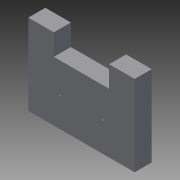
# Autodesk Inventor part: PCB_kon_drzak
Saved by Autodesk Inventor 2015 (Build 190159000, 159)
## iProperties
Created: 2015-12-17
Part Number: PCB_kon_drzak
Material: Generic
Document SubType Name: Modeling
Designer: Turboslimak
Density: 1 g/cm^3
Appearance: Default
Author: Turboslimak
Autodesk Inventor part; units mm, degrees
ref_plane "YZ Plane" through (0, 0, 0) normal (1, 0, 0) x (0, 1, 0)
ref_plane "XZ Plane" through (0, 0, 0) normal (0, 1, 0) x (-1, 0, 0)
ref_plane "XY Plane" through (0, 0, 0) normal (0, 0, 1) x (1, 0, 0)
sketch "Sketch1" plane through (0, 0, 0) normal (0, 1, 0) x (-1, 0, 0)
  line L0 (6.25, 4.75) -> (3.25, 4.75)
  line L1 (3.25, 4.75) -> (3.25, 2.25)
  line L2 (3.25, 2.25) -> (-3.25, 2.25)
  line L3 (-3.25, 2.25) -> (-3.25, 4.75)
  line L4 (-3.25, 4.75) -> (-6.25, 4.75)
  line L5 (6.25, 4.75) -> (6.25, -4.75)
  line L6 (6.25, -4.75) -> (-6.25, -4.75)
  line L7 (-6.25, -4.75) -> (-6.25, 4.75)
  circle A0 centre (2.5, -1.25) radius 0.1
  circle A1 centre (-2.5, -1.25) radius 0.1
  dimension "d0" = 12.5
  dimension "d1" = 9.5
  dimension "d2" = 3
  dimension "d3" = 2.5
  dimension "d4" = 6.5
  dimension "d7" = 0.2
  dimension "d9" = 0.2
  constraints: 16 end point, 3 perpendicular, 2 centre point
  measures "d0" distance of L0.start L4.end
  measures "d1" distance of L5.end L0.start
  measures "d2" distance of L0.start L0.end
  measures "d3" distance of L0.end L1.end
  measures "d4" distance of L1.end L2.end
  measures "d7" diameter of A0
  measures "d9" diameter of A1
extrude "Extrusion1" add sketch "Sketch1" along normal blind 2
body "Solid1"
